Autodesk Inventor part; units mm, degrees
(part 2 of 2)
sketch "Skizze31" plane through (-37.5, 0, 0) normal (-1, 0, 0) x (0, 0, 1)
  circle A0 centre (0, 115) radius 10.1 projected
  line L0 (-0.25, 122.6) -> (0.25, 122.6)
  line L1 (0.25, 122.6) -> (0.25, 127.6)
  line L2 (0.25, 127.6) -> (-0.25, 127.6)
  line L3 (-0.25, 127.6) -> (-0.25, 122.6)
  line L4 (-0.25, 122.6) -> (0.25, 127.6) construction
  line L5 (0.25, 122.6) -> (-0.25, 127.6) construction
  line L6 (-1.5659, 122.4411) -> (-1.0735, 122.528)
  line L7 (-1.0735, 122.528) -> (-1.9418, 127.452)
  line L8 (-1.9418, 127.452) -> (-2.4342, 127.3652)
  line L9 (-2.4342, 127.3652) -> (-1.5659, 122.4411)
  line L10 (-1.5659, 122.4411) -> (-1.9418, 127.452) construction
  line L11 (-1.0735, 122.528) -> (-2.4342, 127.3652) construction
  line L12 (-2.8343, 122.0562) -> (-2.3644, 122.2272)
  line L13 (-2.3644, 122.2272) -> (-4.0745, 126.9256)
  line L14 (-4.0745, 126.9256) -> (-4.5444, 126.7546)
  line L15 (-4.5444, 126.7546) -> (-2.8343, 122.0562)
  line L16 (-2.8343, 122.0562) -> (-4.0745, 126.9256) construction
  line L17 (-2.3644, 122.2272) -> (-4.5444, 126.7546) construction
  line L18 (-4.0165, 121.4568) -> (-3.5835, 121.7068)
  line L19 (-3.5835, 121.7068) -> (-6.0835, 126.0369)
  line L20 (-6.0835, 126.0369) -> (-6.5165, 125.7869)
  line L21 (-6.5165, 125.7869) -> (-4.0165, 121.4568)
  line L22 (-4.0165, 121.4568) -> (-6.0835, 126.0369) construction
  line L23 (-3.5835, 121.7068) -> (-6.5165, 125.7869) construction
  line L24 (-5.0767, 120.6612) -> (-4.6937, 120.9826)
  line L25 (-4.6937, 120.9826) -> (-7.9076, 124.8129)
  line L26 (-7.9076, 124.8129) -> (-8.2906, 124.4915)
  line L27 (-8.2906, 124.4915) -> (-5.0767, 120.6612)
  line L28 (-5.0767, 120.6612) -> (-7.9076, 124.8129) construction
  line L29 (-4.6937, 120.9826) -> (-8.2906, 124.4915) construction
  line L30 (-5.9826, 119.6937) -> (-5.6612, 120.0767)
  line L31 (-5.6612, 120.0767) -> (-9.4915, 123.2906)
  line L32 (-9.4915, 123.2906) -> (-9.8129, 122.9076)
  line L33 (-9.8129, 122.9076) -> (-5.9826, 119.6937)
  line L34 (-5.9826, 119.6937) -> (-9.4915, 123.2906) construction
  line L35 (-5.6612, 120.0767) -> (-9.8129, 122.9076) construction
  line L36 (-6.7068, 118.5835) -> (-6.4568, 119.0165)
  line L37 (-6.4568, 119.0165) -> (-10.7869, 121.5165)
  line L38 (-10.7869, 121.5165) -> (-11.0369, 121.0835)
  line L39 (-11.0369, 121.0835) -> (-6.7068, 118.5835)
  line L40 (-6.7068, 118.5835) -> (-10.7869, 121.5165) construction
  line L41 (-6.4568, 119.0165) -> (-11.0369, 121.0835) construction
  line L42 (-7.2272, 117.3644) -> (-7.0562, 117.8343)
  line L43 (-7.0562, 117.8343) -> (-11.7546, 119.5444)
  line L44 (-11.7546, 119.5444) -> (-11.9256, 119.0745)
  line L45 (-11.9256, 119.0745) -> (-7.2272, 117.3644)
  line L46 (-7.2272, 117.3644) -> (-11.7546, 119.5444) construction
  line L47 (-7.0562, 117.8343) -> (-11.9256, 119.0745) construction
  line L48 (-7.528, 116.0735) -> (-7.4411, 116.5659)
  line L49 (-7.4411, 116.5659) -> (-12.3652, 117.4342)
  line L50 (-12.3652, 117.4342) -> (-12.452, 116.9418)
  line L51 (-12.452, 116.9418) -> (-7.528, 116.0735)
  line L52 (-7.528, 116.0735) -> (-12.3652, 117.4342) construction
  line L53 (-7.4411, 116.5659) -> (-12.452, 116.9418) construction
  line L54 (-7.6, 114.75) -> (-7.6, 115.25)
  line L55 (-7.6, 115.25) -> (-12.6, 115.25)
  line L56 (-12.6, 115.25) -> (-12.6, 114.75)
  line L57 (-12.6, 114.75) -> (-7.6, 114.75)
  line L58 (-7.6, 114.75) -> (-12.6, 115.25) construction
  line L59 (-7.6, 115.25) -> (-12.6, 114.75) construction
  line L60 (-7.4411, 113.4341) -> (-7.528, 113.9265)
  line L61 (-7.528, 113.9265) -> (-12.452, 113.0582)
  line L62 (-12.452, 113.0582) -> (-12.3652, 112.5658)
  line L63 (-12.3652, 112.5658) -> (-7.4411, 113.4341)
  line L64 (-7.4411, 113.4341) -> (-12.452, 113.0582) construction
  line L65 (-7.528, 113.9265) -> (-12.3652, 112.5658) construction
  line L66 (-7.0562, 112.1657) -> (-7.2272, 112.6356)
  line L67 (-7.2272, 112.6356) -> (-11.9256, 110.9255)
  line L68 (-11.9256, 110.9255) -> (-11.7546, 110.4556)
  line L69 (-11.7546, 110.4556) -> (-7.0562, 112.1657)
  line L70 (-7.0562, 112.1657) -> (-11.9256, 110.9255) construction
  line L71 (-7.2272, 112.6356) -> (-11.7546, 110.4556) construction
  line L72 (-6.4568, 110.9835) -> (-6.7068, 111.4165)
  line L73 (-6.7068, 111.4165) -> (-11.0369, 108.9165)
  line L74 (-11.0369, 108.9165) -> (-10.7869, 108.4835)
  line L75 (-10.7869, 108.4835) -> (-6.4568, 110.9835)
  line L76 (-6.4568, 110.9835) -> (-11.0369, 108.9165) construction
  line L77 (-6.7068, 111.4165) -> (-10.7869, 108.4835) construction
  line L78 (-5.6612, 109.9233) -> (-5.9826, 110.3063)
  line L79 (-5.9826, 110.3063) -> (-9.8129, 107.0924)
  line L80 (-9.8129, 107.0924) -> (-9.4915, 106.7094)
  line L81 (-9.4915, 106.7094) -> (-5.6612, 109.9233)
  line L82 (-5.6612, 109.9233) -> (-9.8129, 107.0924) construction
  line L83 (-5.9826, 110.3063) -> (-9.4915, 106.7094) construction
  line L84 (-4.6937, 109.0174) -> (-5.0767, 109.3388)
  line L85 (-5.0767, 109.3388) -> (-8.2906, 105.5085)
  line L86 (-8.2906, 105.5085) -> (-7.9076, 105.1871)
  line L87 (-7.9076, 105.1871) -> (-4.6937, 109.0174)
  line L88 (-4.6937, 109.0174) -> (-8.2906, 105.5085) construction
  line L89 (-5.0767, 109.3388) -> (-7.9076, 105.1871) construction
  line L90 (-3.5835, 108.2932) -> (-4.0165, 108.5432)
  line L91 (-4.0165, 108.5432) -> (-6.5165, 104.2131)
  line L92 (-6.5165, 104.2131) -> (-6.0835, 103.9631)
  line L93 (-6.0835, 103.9631) -> (-3.5835, 108.2932)
  line L94 (-3.5835, 108.2932) -> (-6.5165, 104.2131) construction
  line L95 (-4.0165, 108.5432) -> (-6.0835, 103.9631) construction
  line L96 (-2.3644, 107.7728) -> (-2.8343, 107.9438)
  line L97 (-2.8343, 107.9438) -> (-4.5444, 103.2454)
  line L98 (-4.5444, 103.2454) -> (-4.0745, 103.0744)
  line L99 (-4.0745, 103.0744) -> (-2.3644, 107.7728)
  line L100 (-2.3644, 107.7728) -> (-4.5444, 103.2454) construction
  line L101 (-2.8343, 107.9438) -> (-4.0745, 103.0744) construction
  line L102 (-1.0735, 107.472) -> (-1.5659, 107.5589)
  line L103 (-1.5659, 107.5589) -> (-2.4342, 102.6348)
  line L104 (-2.4342, 102.6348) -> (-1.9418, 102.548)
  line L105 (-1.9418, 102.548) -> (-1.0735, 107.472)
  line L106 (-1.0735, 107.472) -> (-2.4342, 102.6348) construction
  line L107 (-1.5659, 107.5589) -> (-1.9418, 102.548) construction
  line L108 (0.25, 107.4) -> (-0.25, 107.4)
  line L109 (-0.25, 107.4) -> (-0.25, 102.4)
  line L110 (-0.25, 102.4) -> (0.25, 102.4)
  line L111 (0.25, 102.4) -> (0.25, 107.4)
  line L112 (0.25, 107.4) -> (-0.25, 102.4) construction
  line L113 (-0.25, 107.4) -> (0.25, 102.4) construction
  line L114 (1.5659, 107.5589) -> (1.0735, 107.472)
  line L115 (1.0735, 107.472) -> (1.9418, 102.548)
  line L116 (1.9418, 102.548) -> (2.4342, 102.6348)
  line L117 (2.4342, 102.6348) -> (1.5659, 107.5589)
  line L118 (1.5659, 107.5589) -> (1.9418, 102.548) construction
  line L119 (1.0735, 107.472) -> (2.4342, 102.6348) construction
  line L120 (2.8343, 107.9438) -> (2.3644, 107.7728)
  line L121 (2.3644, 107.7728) -> (4.0745, 103.0744)
  line L122 (4.0745, 103.0744) -> (4.5444, 103.2454)
  line L123 (4.5444, 103.2454) -> (2.8343, 107.9438)
  line L124 (2.8343, 107.9438) -> (4.0745, 103.0744) construction
  line L125 (2.3644, 107.7728) -> (4.5444, 103.2454) construction
  line L126 (4.0165, 108.5432) -> (3.5835, 108.2932)
  line L127 (3.5835, 108.2932) -> (6.0835, 103.9631)
  line L128 (6.0835, 103.9631) -> (6.5165, 104.2131)
  line L129 (6.5165, 104.2131) -> (4.0165, 108.5432)
  line L130 (4.0165, 108.5432) -> (6.0835, 103.9631) construction
  line L131 (3.5835, 108.2932) -> (6.5165, 104.2131) construction
  line L132 (5.0767, 109.3388) -> (4.6937, 109.0174)
  line L133 (4.6937, 109.0174) -> (7.9076, 105.1871)
  line L134 (7.9076, 105.1871) -> (8.2906, 105.5085)
  line L135 (8.2906, 105.5085) -> (5.0767, 109.3388)
  line L136 (5.0767, 109.3388) -> (7.9076, 105.1871) construction
  line L137 (4.6937, 109.0174) -> (8.2906, 105.5085) construction
  line L138 (5.9826, 110.3063) -> (5.6612, 109.9233)
  line L139 (5.6612, 109.9233) -> (9.4915, 106.7094)
  line L140 (9.4915, 106.7094) -> (9.8129, 107.0924)
  line L141 (9.8129, 107.0924) -> (5.9826, 110.3063)
  line L142 (5.9826, 110.3063) -> (9.4915, 106.7094) construction
  line L143 (5.6612, 109.9233) -> (9.8129, 107.0924) construction
  line L144 (6.7068, 111.4165) -> (6.4568, 110.9835)
  line L145 (6.4568, 110.9835) -> (10.7869, 108.4835)
  line L146 (10.7869, 108.4835) -> (11.0369, 108.9165)
  line L147 (11.0369, 108.9165) -> (6.7068, 111.4165)
  line L148 (6.7068, 111.4165) -> (10.7869, 108.4835) construction
  line L149 (6.4568, 110.9835) -> (11.0369, 108.9165) construction
  line L150 (7.2272, 112.6356) -> (7.0562, 112.1657)
  line L151 (7.0562, 112.1657) -> (11.7546, 110.4556)
  line L152 (11.7546, 110.4556) -> (11.9256, 110.9255)
  line L153 (11.9256, 110.9255) -> (7.2272, 112.6356)
  line L154 (7.2272, 112.6356) -> (11.7546, 110.4556) construction
  line L155 (7.0562, 112.1657) -> (11.9256, 110.9255) construction
  line L156 (7.528, 113.9265) -> (7.4411, 113.4341)
  line L157 (7.4411, 113.4341) -> (12.3652, 112.5658)
  line L158 (12.3652, 112.5658) -> (12.452, 113.0582)
  line L159 (12.452, 113.0582) -> (7.528, 113.9265)
  line L160 (7.528, 113.9265) -> (12.3652, 112.5658) construction
  line L161 (7.4411, 113.4341) -> (12.452, 113.0582) construction
  line L162 (7.6, 115.25) -> (7.6, 114.75)
  line L163 (7.6, 114.75) -> (12.6, 114.75)
  line L164 (12.6, 114.75) -> (12.6, 115.25)
  line L165 (12.6, 115.25) -> (7.6, 115.25)
  line L166 (7.6, 115.25) -> (12.6, 114.75) construction
  line L167 (7.6, 114.75) -> (12.6, 115.25) construction
  line L168 (7.4411, 116.5659) -> (7.528, 116.0735)
  line L169 (7.528, 116.0735) -> (12.452, 116.9418)
  line L170 (12.452, 116.9418) -> (12.3652, 117.4342)
  line L171 (12.3652, 117.4342) -> (7.4411, 116.5659)
  line L172 (7.4411, 116.5659) -> (12.452, 116.9418) construction
  line L173 (7.528, 116.0735) -> (12.3652, 117.4342) construction
  line L174 (7.0562, 117.8343) -> (7.2272, 117.3644)
  line L175 (7.2272, 117.3644) -> (11.9256, 119.0745)
  line L176 (11.9256, 119.0745) -> (11.7546, 119.5444)
  line L177 (11.7546, 119.5444) -> (7.0562, 117.8343)
  line L178 (7.0562, 117.8343) -> (11.9256, 119.0745) construction
  line L179 (7.2272, 117.3644) -> (11.7546, 119.5444) construction
  line L180 (6.4568, 119.0165) -> (6.7068, 118.5835)
  line L181 (6.7068, 118.5835) -> (11.0369, 121.0835)
  line L182 (11.0369, 121.0835) -> (10.7869, 121.5165)
  line L183 (10.7869, 121.5165) -> (6.4568, 119.0165)
  line L184 (6.4568, 119.0165) -> (11.0369, 121.0835) construction
  line L185 (6.7068, 118.5835) -> (10.7869, 121.5165) construction
  line L186 (5.6612, 120.0767) -> (5.9826, 119.6937)
  line L187 (5.9826, 119.6937) -> (9.8129, 122.9076)
  line L188 (9.8129, 122.9076) -> (9.4915, 123.2906)
  line L189 (9.4915, 123.2906) -> (5.6612, 120.0767)
  line L190 (5.6612, 120.0767) -> (9.8129, 122.9076) construction
  line L191 (5.9826, 119.6937) -> (9.4915, 123.2906) construction
  line L192 (4.6937, 120.9826) -> (5.0767, 120.6612)
  line L193 (5.0767, 120.6612) -> (8.2906, 124.4915)
  line L194 (8.2906, 124.4915) -> (7.9076, 124.8129)
  line L195 (7.9076, 124.8129) -> (4.6937, 120.9826)
  line L196 (4.6937, 120.9826) -> (8.2906, 124.4915) construction
  line L197 (5.0767, 120.6612) -> (7.9076, 124.8129) construction
  line L198 (3.5835, 121.7068) -> (4.0165, 121.4568)
  line L199 (4.0165, 121.4568) -> (6.5165, 125.7869)
  line L200 (6.5165, 125.7869) -> (6.0835, 126.0369)
  line L201 (6.0835, 126.0369) -> (3.5835, 121.7068)
  line L202 (3.5835, 121.7068) -> (6.5165, 125.7869) construction
  line L203 (4.0165, 121.4568) -> (6.0835, 126.0369) construction
  line L204 (2.3644, 122.2272) -> (2.8343, 122.0562)
  line L205 (2.8343, 122.0562) -> (4.5444, 126.7546)
  line L206 (4.5444, 126.7546) -> (4.0745, 126.9256)
  line L207 (4.0745, 126.9256) -> (2.3644, 122.2272)
  line L208 (2.3644, 122.2272) -> (4.5444, 126.7546) construction
  line L209 (2.8343, 122.0562) -> (4.0745, 126.9256) construction
  line L210 (1.0735, 122.528) -> (1.5659, 122.4411)
  line L211 (1.5659, 122.4411) -> (2.4342, 127.3652)
  line L212 (2.4342, 127.3652) -> (1.9418, 127.452)
  line L213 (1.9418, 127.452) -> (1.0735, 122.528)
  line L214 (1.0735, 122.528) -> (2.4342, 127.3652) construction
  line L215 (1.5659, 122.4411) -> (1.9418, 127.452) construction
  line L216 (-0.25, 100) -> (0.25, 100)
  line L217 (0.25, 100) -> (0.25, 130)
  line L218 (0.25, 130) -> (-0.25, 130)
  line L219 (-0.25, 130) -> (-0.25, 100)
  line L220 (-0.25, 100) -> (0.25, 130) construction
  line L221 (0.25, 100) -> (-0.25, 130) construction
  line L222 (15, 114.75) -> (-15, 114.75)
  line L223 (-15, 114.75) -> (-15, 115.25)
  line L224 (-15, 115.25) -> (15, 115.25)
  line L225 (15, 115.25) -> (15, 114.75)
  line L226 (15, 114.75) -> (-15, 115.25) construction
  line L227 (-15, 114.75) -> (15, 115.25) construction
  point P0 (0, 0)
  point P1 (0, 125.1)
  point P2 (-1.7538, 124.9466)
  point P3 (-3.4544, 124.4909)
  point P4 (-5.05, 123.7469)
  point P5 (-6.4922, 122.737)
  point P6 (-7.737, 121.4922)
  point P7 (-8.7469, 120.05)
  point P8 (-9.4909, 118.4544)
  point P9 (-9.9466, 116.7538)
  point P10 (-10.1, 115)
  point P11 (-9.9466, 113.2462)
  point P12 (-9.4909, 111.5456)
  point P13 (-8.7469, 109.95)
  point P14 (-7.737, 108.5078)
  point P15 (-6.4922, 107.263)
  point P16 (-5.05, 106.2531)
  point P17 (-3.4544, 105.5091)
  point P18 (-1.7538, 105.0534)
  point P19 (0, 104.9)
  point P20 (1.7538, 105.0534)
  point P21 (3.4544, 105.5091)
  point P22 (5.05, 106.2531)
  point P23 (6.4922, 107.263)
  point P24 (7.737, 108.5078)
  point P25 (8.7469, 109.95)
  point P26 (9.4909, 111.5456)
  point P27 (9.9466, 113.2462)
  point P28 (10.1, 115)
  point P29 (9.9466, 116.7538)
  point P30 (9.4909, 118.4544)
  point P31 (8.7469, 120.05)
  point P32 (7.737, 121.4922)
  point P33 (6.4922, 122.737)
  point P34 (5.05, 123.7469)
  point P35 (3.4544, 124.4909)
  point P36 (1.7538, 124.9466)
  dimension "d143" = 0.5
  dimension "d144" = 5
  dimension "d147" = 360
  dimension "d149" = 0.5
  dimension "d150" = 30
  constraints: 456 end point, 76 midpoint, 6 parallel, 3 horizontal, 3 perpendicular, 1 vertical alignment, 398 other
  measures "d143" distance of L2.end L1.end
  measures "d144" distance of L1.end L0.end
  measures "d149" distance of L218.end L217.end
  measures "d150" distance of L217.end L216.end
extrude "Extrusion25" cut sketch "Skizze31" against normal blind 0.5 contours A0 L163 L162 L165 | A0 L165 L164 L163 | L169 L168 L171 A0 | A0 L171 L170 L169 | L224 L225 L222 L164 | L162 L222 L217 L224 | L159 L158 L157 A0 | A0 L157 L156 L159 | L224 L219 L0 L217 | L217 L222 L219 L224 | L217 L108 L219 L222 | L175 L174 L177 A0 | A0 L177 L176 L175 | L0 L3 A0 L1 | L219 L222 L54 L224 | L153 L152 L151 A0 | A0 L151 L150 L153 | L111 A0 L109 L108 | A0 L3 L2 L1 | L54 L57 A0 L55 | L111 L110 L109 A0 | L181 L180 L183 A0 | A0 L183 L182 L181 | L213 L212 L211 A0 | A0 L211 L210 L213 | L2 L219 L218 L217 | A0 L57 L56 L55 | L147 L146 L145 A0 | A0 L145 L144 L147 | L115 L114 L117 A0 | A0 L117 L116 L115 | L217 L216 L219 L110 | L7 L6 L9 A0 | A0 L9 L8 L7 | L51 L50 L49 A0 | A0 L49 L48 L51 | L56 L222 L223 L224 | L105 L104 L103 A0 | A0 L103 L102 L105 | L61 L60 L63 A0 | A0 L63 L62 L61 | L187 L186 L189 A0 | A0 L189 L188 L187 | L207 L206 L205 A0 | A0 L205 L204 L207 | L141 L140 L139 A0 | A0 L139 L138 L141 | L121 L120 L123 A0 | A0 L123 L122 L121 | L13 L12 L15 A0 | A0 L15 L14 L13 | L45 L44 L43 A0 | A0 L43 L42 L45 | L99 L98 L97 A0 | A0 L97 L96 L99 | L67 L66 L69 A0 | A0 L69 L68 L67 | L193 L192 L195 A0 | A0 L195 L194 L193 | L201 L200 L199 A0 | A0 L199 L198 L201 | L135 L134 L133 A0 | A0 L133 L132 L135 | L127 L126 L129 A0 | A0 L129 L128 L127 | L19 L18 L21 A0 | A0 L21 L20 L19 | L39 L38 L37 A0 | A0 L37 L36 L39 | L93 L92 L91 A0 | A0 L91 L90 L93 | L73 L72 L75 A0 | A0 L75 L74 L73 | L25 L24 L27 A0 | A0 L27 L26 L25 | L33 L32 L31 A0 | A0 L31 L30 L33 | L87 L86 L85 A0 | A0 L85 L84 L87 | L79 L78 L81 A0 | A0 L81 L80 L79
sketch "Skizze32" plane through (-37.5, 0, 0) normal (-1, 0, 0) x (0, 0, 1)
  line L0 (-18.0821, 133.4662) -> (-6.8598, 133.4662) construction
  line L1 (-6.8598, 133.4662) -> (-6.8598, 125.6271) construction
  line L2 (-6.8598, 125.6271) -> (-18.0821, 125.6271) construction
  line L3 (-18.0821, 125.6271) -> (-18.0821, 133.4662) construction
  line L4 (-15.8442, 129.8953) -> (-17.5517, 129.8953)
  line L5 (-17.5517, 129.8953) -> (-17.5517, 130.2526)
  line L6 (-17.5517, 130.2526) -> (-16.9163, 130.2526)
  line L7 (-16.9163, 130.2526) -> (-16.9163, 132.5983)
  line L8 (-16.9163, 132.5983) -> (-17.5517, 132.5983)
  line L9 (-17.5517, 132.5983) -> (-17.5517, 132.9188)
  spline S0 degree 2 poles (-17.5517, 132.9188) (-17.1915, 132.9188) (-16.8511, 133.123) (-16.8284, 133.4066) knots 0 0 0 1 2 2 2
  line L10 (-16.8284, 133.4066) -> (-16.4654, 133.4066)
  line L11 (-16.4654, 133.4066) -> (-16.4654, 130.2526)
  line L12 (-16.4654, 130.2526) -> (-15.8442, 130.2526)
  line L13 (-15.8442, 130.2526) -> (-15.8442, 129.8953)
  spline S1 degree 2 poles (-13.0221, 131.6453) (-13.0221, 130.7036) (-13.5695, 129.8215) (-14.1396, 129.8215) knots 0 0 0 1 2 2 2
  spline S2 degree 2 poles (-14.1396, 129.8215) (-14.7182, 129.8215) (-15.2599, 130.7206) (-15.2599, 131.6424) knots 0 0 0 1 2 2 2
  spline S3 degree 2 poles (-15.2599, 131.6424) (-15.2599, 132.5898) (-14.7125, 133.4662) (-14.1396, 133.4662) knots 0 0 0 1 2 2 2
  spline S4 degree 2 poles (-14.1396, 133.4662) (-13.5638, 133.4662) (-13.0221, 132.5586) (-13.0221, 131.6453) knots 0 0 0 1 2 2 2
  spline S5 degree 2 poles (-13.6234, 130.5788) (-13.5553, 130.7518) (-13.4986, 131.2851) (-13.4986, 131.6453) knots 0 0 0 1 2 2 2
  spline S6 degree 2 poles (-13.4986, 131.6453) (-13.4986, 132.0055) (-13.5553, 132.5359) (-13.6262, 132.7146) knots 0 0 0 1 2 2 2
  spline S7 degree 2 poles (-13.6262, 132.7146) (-13.6971, 132.8932) (-13.9439, 133.0776) (-14.1396, 133.0776) knots 0 0 0 1 2 2 2
  spline S8 degree 2 poles (-14.1396, 133.0776) (-14.3353, 133.0776) (-14.5877, 132.8932) (-14.6615, 132.7089) knots 0 0 0 1 2 2 2
  spline S9 degree 2 poles (-14.6615, 132.7089) (-14.7324, 132.5302) (-14.7834, 131.9856) (-14.7834, 131.6424) knots 0 0 0 1 2 2 2
  spline S10 degree 2 poles (-14.7834, 131.6424) (-14.7834, 131.2737) (-14.7381, 130.7802) (-14.6643, 130.5873) knots 0 0 0 1 2 2 2
  spline S11 degree 2 poles (-14.6643, 130.5873) (-14.5962, 130.4058) (-14.3438, 130.2101) (-14.1396, 130.2101) knots 0 0 0 1 2 2 2
  spline S12 degree 2 poles (-14.1396, 130.2101) (-13.9467, 130.2101) (-13.6943, 130.3945) (-13.6234, 130.5788) knots 0 0 0 1 2 2 2
  spline S13 degree 2 poles (-10.8013, 132.5614) (-10.8013, 132.1842) (-11.3175, 131.668) (-11.6947, 131.668) knots 0 0 0 1 2 2 2
  spline S14 degree 2 poles (-11.6947, 131.668) (-12.0691, 131.668) (-12.591, 132.1813) (-12.591, 132.5614) knots 0 0 0 1 2 2 2
  spline S15 degree 2 poles (-12.591, 132.5614) (-12.591, 132.9386) (-12.0748, 133.4548) (-11.6947, 133.4548) knots 0 0 0 1 2 2 2
  spline S16 degree 2 poles (-11.6947, 133.4548) (-11.3175, 133.4548) (-10.8013, 132.9386) (-10.8013, 132.5614) knots 0 0 0 1 2 2 2
  spline S17 degree 2 poles (-11.17, 132.5614) (-11.17, 132.7883) (-11.4706, 133.0975) (-11.6947, 133.0975) knots 0 0 0 1 2 2 2
  spline S18 degree 2 poles (-11.6947, 133.0975) (-11.9216, 133.0975) (-12.2223, 132.7883) (-12.2223, 132.5614) knots 0 0 0 1 2 2 2
  spline S19 degree 2 poles (-12.2223, 132.5614) (-12.2223, 132.3317) (-11.9159, 132.0253) (-11.6947, 132.0253) knots 0 0 0 1 2 2 2
  spline S20 degree 2 poles (-11.6947, 132.0253) (-11.4706, 132.0253) (-11.17, 132.3373) (-11.17, 132.5614) knots 0 0 0 1 2 2 2
  point P0 (0, 0)
  constraints: 2 other
extrude "Extrusion26" cut sketch "Skizze32" against normal blind 0.5
sketch "Skizze33" plane through (-37.5, 0, 0) normal (-1, 0, 0) x (0, 0, 1)
  line L0 (2.65, 16.3048) -> (2.65, 66.6048) projected
  line L1 (7.5, 41.7048) -> (-7.5, 41.7048)
  line L2 (-7.5, 41.7048) -> (-7.5, 41.2048)
  line L3 (-7.5, 41.2048) -> (7.5, 41.2048)
  line L4 (7.5, 41.2048) -> (7.5, 41.7048)
  line L5 (7.5, 41.7048) -> (-7.5, 41.2048) construction
  line L6 (-7.5, 41.7048) -> (7.5, 41.2048) construction
  point P0 (0, 0)
  point P1 (0, 41.4548)
  dimension "d155" = 0.5
  constraints: 12 end point, 2 midpoint, 2 parallel, 1 horizontal, 1 perpendicular
  measures "d155" distance of L2.end L1.end
extrude "Extrusion27" cut sketch "Skizze33" against normal blind 0.5
sketch "Skizze34" plane through (-37.5, 135, 0) normal (0, 1, 0) x (1, 0, 0)
  line L0 (37.75, 5) -> (37.25, 5)
  line L1 (37.25, 5) -> (37.25, -5)
  line L2 (37.25, -5) -> (37.75, -5)
  line L3 (37.75, -5) -> (37.75, 5)
  line L4 (37.75, 5) -> (37.25, -5) construction
  line L5 (37.25, 5) -> (37.75, -5) construction
  line L6 (32.5, 0.25) -> (42.5, 0.25)
  line L7 (42.5, 0.25) -> (42.5, -0.25)
  line L8 (42.5, -0.25) -> (32.5, -0.25)
  line L9 (32.5, -0.25) -> (32.5, 0.25)
  line L10 (32.5, 0.25) -> (42.5, -0.25) construction
  line L11 (42.5, 0.25) -> (32.5, -0.25) construction
  point P0 (37.5, 0)
  dimension "d158" = 10
  dimension "d159" = 10
  dimension "d160" = 0.5
  constraints: 24 end point, 4 midpoint, 4 parallel, 2 horizontal, 2 perpendicular
  measures "d158" distance of L1.end L0.end
  measures "d159" distance of L7.end L8.end
  measures "d160" distance of L6.end L7.end
extrude "Extrusion28" cut sketch "Skizze34" against normal blind 0.5
sketch "Skizze35" plane through (-37.5, 135, -20) normal (0, 1, 0) x (1, 0, 0)
  line L0 (32.5, -12.25) -> (42.5, -12.25)
  line L1 (42.5, -12.25) -> (42.5, -12.75)
  line L2 (42.5, -12.75) -> (32.5, -12.75)
  line L3 (32.5, -12.75) -> (32.5, -12.25)
  line L4 (0, -12.5) -> (75, -12.5) projected
  line L5 (32.5, -12.25) -> (42.5, -12.75) construction
  line L6 (42.5, -12.25) -> (32.5, -12.75) construction
  line L7 (37.75, -15) -> (37.75, -19.75) projected
  line L8 (37.25, -6.4506) -> (37.75, -6.4506)
  line L9 (37.75, -6.4506) -> (37.75, -18.5494)
  line L10 (37.75, -18.5494) -> (37.25, -18.5494)
  line L11 (37.25, -18.5494) -> (37.25, -6.4506)
  line L12 (35.9, -12.5) -> (39.1, -12.5) projected
  line L13 (37.25, -6.4506) -> (37.75, -18.5494) construction
  line L14 (37.75, -6.4506) -> (37.25, -18.5494) construction
  point P0 (37.5, -20)
  point P1 (37.5, -12.5)
  point P2 (37.5, -12.5)
  dimension "d163" = 10
  dimension "d164" = 0.5
  constraints: 24 end point, 6 midpoint, 4 parallel, 2 horizontal, 2 perpendicular, 1 point on line
  measures "d163" distance of L1.end L2.end
  measures "d164" distance of L0.end L1.end
extrude "Extrusion29" cut sketch "Skizze35" against normal blind 0.5
